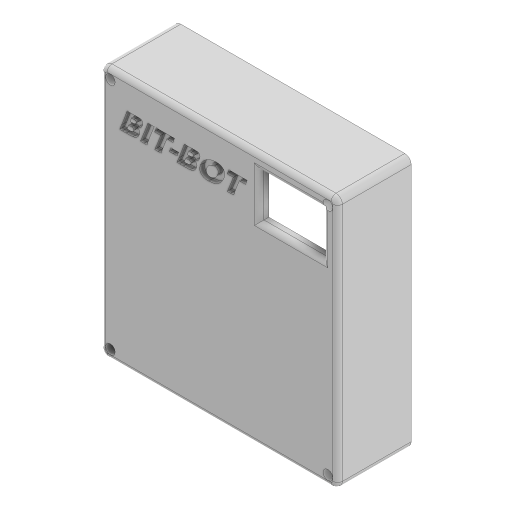
# Autodesk Inventor part: bit bot battery pack
Saved by Autodesk Inventor 2024 (Build 280153000, 153)
## iProperties
Created: 2024-01-11
Part Number: bit bot battery pack
Material: Generic
Document SubType Name: Modeling
Designer: chris
Density: 1 g/cm^3
Appearance: Default
Author: chris
Autodesk Inventor part; units mm, degrees
ref_plane "YZ Plane" through (0, 0, 0) normal (1, 0, 0) x (0, 1, 0)
ref_plane "XZ Plane" through (0, 0, 0) normal (0, 1, 0) x (-1, 0, 0)
ref_plane "XY Plane" through (0, 0, 0) normal (0, 0, 1) x (1, 0, 0)
sketch "Sketch2" plane through (0, 0, 0) normal (0, 0, 1) x (1, 0, 0)
  line L0 (0, -40) -> (0, -15)
  line L1 (0, -15) -> (-34, -15)
  line L2 (-34, -15) -> (-34, 58)
  line L3 (-34, 58) -> (34, 58)
  line L4 (34, 58) -> (34, -15)
  line L5 (34, -15) -> (0, -15)
  circle A0 centre (-34, 58) radius 1.5
  circle A1 centre (34, 58) radius 1.5
  circle A2 centre (-34, -15) radius 1.5
  circle A3 centre (34, -15) radius 1.5
  line L6 (32.5, 56.5) -> (-32.5, 56.5)
  line L7 (-32.5, 56.5) -> (-32.5, -13.5)
  line L8 (-32.5, -13.5) -> (0, -13.5)
  line L9 (0, -13.5) -> (32.5, -13.5)
  line L10 (32.5, -13.5) -> (32.5, 56.5)
  line L11 (37, -18) -> (37, 61)
  line L12 (37, 61) -> (-37, 61)
  line L13 (-37, 61) -> (-37, -18)
  line L14 (-37, -18) -> (0, -18)
  line L15 (0, -18) -> (37, -18)
  point P0 (0, 0)
  dimension "d0" = 25
  dimension "d1" = 34
  dimension "d3" = 68
  dimension "d4" = 3
  dimension "d5" = 3
  dimension "d6" = 3
  dimension "d11" = 1.5
  dimension "d13" = 3
  constraints: 32 end point, 13 perpendicular, 4 centre point, 4 coincident, 1 point on line, 1 vertical, 8 other
  measures "d0" distance of L0.start L0.end
  measures "d1" distance of L0.end L1.end
  measures "d3" distance of L2.end L3.end
  measures "d4" diameter of A0
  measures "d5" diameter of A1
  measures "d6" diameter of A2
  measures "d11" distance between parallel lines of L3 L6
  measures "d13" distance between parallel lines of L4 L11
extrude "Extrusion1" add sketch "Sketch2" along normal blind 20 contours L1 A2 L2 A0 L3 A1 L4 A3 L5 | L15 L14 L13 L12 L11
fillet "Fillet1" radius 2 4 edges at (37, -18, 10) (37, 61, 10) (-37, 61, 10) (-37, -18, 10)
sketch "Sketch3" plane through (0, 0, 20) normal (0, 0, 1) x (1, 0, 0)
  arc A0 (-37, -16) -> (-35, -18) centre (-35, -16) ccw projected
  line L0 (-35, -18) -> (35, -18) projected
  arc A1 (35, -18) -> (37, -16) centre (35, -16) ccw projected
  line L1 (37, -16) -> (37, 59) projected
  arc A2 (37, 59) -> (35, 61) centre (35, 59) ccw projected
  line L2 (35, 61) -> (-35, 61) projected
  arc A3 (-35, 61) -> (-37, 59) centre (-35, 59) ccw projected
  line L3 (-37, 59) -> (-37, -16) projected
  circle A4 centre (34, -15) radius 1.5 projected
  circle A5 centre (-34, -15) radius 1.5 projected
  circle A6 centre (-34, 58) radius 1.5 projected
  line L4 (32.5, 56.5) -> (32.5, -13.5) projected
  line L5 (32.5, -13.5) -> (-32.5, -13.5) projected
  line L6 (-32.5, -13.5) -> (-32.5, 56.5) projected
  line L7 (-32.5, 56.5) -> (32.5, 56.5) projected
  circle A7 centre (34, 58) radius 1.5 projected
  point P0 (0, 0)
extrude "Extrusion2" add sketch "Sketch3" along normal blind 3 contours L3 A3 L2 A2 L1 A1 L0 A0 | L4 L5 L6 L7
fillet "Fillet2" radius 1.5 8 edges at (36.4142, 60.4142, 23) (0, 61, 23) (-36.4142, 60.4142, 23) (-37, 21.5, 23) (-36.4142, -17.4142, 23) (0, -18, 23) (36.4142, -17.4142, 23) (37, 21.5, 23)
sketch "Sketch4" plane through (0, 0, 20) normal (0, 0, -1) x (-1, 0, 0)
  line L0 (-32.5, 56.5) -> (-32.5, -13.5) projected
  line L1 (-32.5, 56.5) -> (-12.5, 56.5)
  line L2 (32.5, 56.5) -> (-32.5, 56.5) projected
  line L3 (-12.5, 56.5) -> (-12.5, 42.5)
  line L4 (-12.5, 42.5) -> (-32.5, 42.5)
  point P0 (0, 0)
  dimension "d18" = 20
  dimension "d19" = 14
  constraints: 6 end point, 2 perpendicular, 1 point on line
  measures "d18" distance of L0.start L1.end
  measures "d19" distance of L1.end L3.end
extrude "Extrusion3" cut sketch "Sketch4" against normal blind 3
fillet "Fillet3" radius 1.5 4 edges at (12.5, 49.5, 23) (22.5, 56.5, 23) (32.5, 49.5, 23) (22.5, 42.5, 23)
sketch "Sketch7" plane through (0, 0, 0) normal (0, 0, -1) x (-1, 0, 0)
  line L0 (32.5, -13.5) -> (32.5, 56.5) projected
  line L1 (32.5, 56.5) -> (27.5, 56.5)
  line L2 (32.5, 56.5) -> (-32.5, 56.5) projected
  line L3 (27.5, 56.5) -> (29.5, 56.5)
  line L4 (29.5, 56.5) -> (29.5, 58.5)
  line L5 (29.5, 58.5) -> (25.5, 58.5)
  line L6 (25.5, 58.5) -> (25.5, 56.5)
  line L7 (29.5, 58.5) -> (31, 58.5)
  line L8 (31, 58.5) -> (31, 56.5)
  line L9 (25.5, 58.5) -> (24, 58.5)
  line L10 (24, 58.5) -> (24, 56.5)
  line L11 (0, 56.5) -> (0, 48.9008)
  line L12 (-32.5, 56.5) -> (-27.5, 56.5)
  line L13 (-32.5, 56.5) -> (32.5, 56.5)
  line L14 (-27.5, 56.5) -> (-29.5, 56.5)
  line L15 (-29.5, 56.5) -> (-29.5, 58.5)
  line L16 (-29.5, 58.5) -> (-25.5, 58.5)
  line L17 (-25.5, 58.5) -> (-25.5, 56.5)
  line L18 (-29.5, 58.5) -> (-31, 58.5)
  line L19 (-31, 58.5) -> (-31, 56.5)
  line L20 (-25.5, 58.5) -> (-24, 58.5)
  line L21 (-24, 58.5) -> (-24, 56.5)
  line L22 (24, 58.5) -> (-24, 58.5)
  point P0 (0, 0)
  dimension "d44" = 5
  dimension "d45" = 2
  dimension "d46" = 2
  dimension "d47" = 4
  dimension "d48" = 1.5
  dimension "d49" = 1.5
  constraints: 42 end point, 14 point on line, 11 symmetric about line, 4 perpendicular, 2 vertical, 1 midpoint, 1 parallel
  measures "d44" distance of L0.end L1.end
  measures "d45" distance of L1.end L3.end
  measures "d46" distance of L3.end L4.end
  measures "d47" distance of L4.end L5.end
  measures "d48" distance of L4.end L7.end
  measures "d49" distance of L5.end L9.end
extrude "Extrusion6" cut sketch "Sketch7" against normal up to surface (20 mm away)
fillet "Fillet5" radius 1.5 4 edges at (31, 58.5, 10) (31, 56.5, 10) (-31, 58.5, 10) (-31, 56.5, 10)
sketch "Sketch12" plane through (-35, -18, 0) normal (0, -1, 0) x (1, 0, 0)
  line L0 (1, 23) -> (69, 23) projected
  line L1 (35, 11.5) -> (17.5, 11.5)
  line L2 (17.5, 11.5) -> (52.5, 11.5)
  circle A0 centre (17.5, 11.5) radius 6
  circle A1 centre (52.5, 11.5) radius 6
  line L3 (35, 11.5) -> (35, 13)
  line L4 (35, 13) -> (17.5, 13)
  line L5 (17.5, 13) -> (53.6469, 13)
  line L6 (35, 11.5) -> (35, 10)
  line L7 (35, 10) -> (18.6171, 10)
  line L8 (18.6171, 10) -> (53.6469, 10)
  point P0 (35, 0)
  dimension "d60" = 17.5
  dimension "d61" = 35
  dimension "d62" = 12
  dimension "d63" = 12
  dimension "d68" = 1.5
  dimension "d69" = 1.5
  constraints: 16 end point, 3 perpendicular, 3 point on line, 2 centre point, 2 coincident, 1 horizontal, 1 vertical
  measures "d60" distance of L1.start L1.end
  measures "d61" distance of L1.end L2.end
  measures "d62" diameter of A0
  measures "d63" diameter of A1
  measures "d68" distance of L1.start L3.end
  measures "d69" distance of L1.start L6.end
extrude "Extrusion8" cut sketch "Sketch12" against normal blind 1 contours A0 | A1
sketch "Sketch13" plane through (0, 0, 23) normal (0, 0, 1) x (1, 0, 0)
  line L0 (-31.5692, 52.222) -> (-1.4752, 52.222) construction
  line L1 (-1.4752, 52.222) -> (-1.4752, 34.913) construction
  line L2 (-1.4752, 34.913) -> (-31.5692, 34.913) construction
  line L3 (-31.5692, 34.913) -> (-31.5692, 52.222) construction
  spline S0 degree 2 poles (-31.1035, 46.0094) (-30.6737, 46.992) (-30.4536, 47.5549) knots 0 0 0 1 1 1
  spline S1 degree 2 poles (-30.4536, 47.5549) (-30.1466, 48.3225) (-29.1487, 51.004) (-28.9593, 51.5567) knots 0 0 0 1 2 2 2
  spline S2 degree 2 poles (-28.9593, 51.5567) (-28.8928, 51.7512) (-28.7751, 52.1094) knots 0 0 0 1 1 1
  spline S3 degree 2 poles (-28.7751, 52.1094) (-28.1866, 52.0941) (-27.8386, 52.0941) knots 0 0 0 1 1 1
  spline S4 degree 2 poles (-27.8386, 52.0941) (-27.3525, 52.0941) (-26.0424, 52.135) (-25.5767, 52.135) knots 0 0 0 1 2 2 2
  spline S5 degree 2 poles (-25.5767, 52.135) (-25.0189, 52.135) (-24.7937, 52.1043) knots 0 0 0 1 1 1
  spline S6 degree 2 poles (-24.7937, 52.1043) (-24.4918, 52.0634) (-24.0926, 51.8587) (-23.9903, 51.7051) knots 0 0 0 1 2 2 2
  spline S7 degree 2 poles (-23.9903, 51.7051) (-23.8726, 51.5311) (-23.8624, 51.2804) knots 0 0 0 1 1 1
  spline S8 degree 2 poles (-23.8624, 51.2804) (-23.847, 50.9938) (-23.9596, 50.6663) knots 0 0 0 1 1 1
  spline S9 degree 2 poles (-23.9596, 50.6663) (-24.0466, 50.4104) (-24.3332, 49.9499) (-24.6914, 49.5865) (-25.0701, 49.346) (-25.3976, 49.2129) (-25.6586, 49.1464) knots 0 0 0 1 2 3 4 5 5 5
  spline S10 degree 2 poles (-25.6586, 49.1464) (-25.4334, 49.1055) (-25.1827, 49.0031) (-24.9319, 48.7728) (-24.7988, 48.4146) (-24.8193, 47.9745) (-24.9012, 47.7289) knots 0 0 0 1 2 3 4 5 5 5
  spline S11 degree 2 poles (-24.9012, 47.7289) (-25.0189, 47.386) (-25.4436, 46.7873) (-25.72, 46.5723) knots 0 0 0 1 2 2 2
  spline S12 degree 2 poles (-25.72, 46.5723) (-25.9503, 46.3881) (-26.5848, 46.1322) (-26.8868, 46.0811) knots 0 0 0 1 2 2 2
  spline S13 degree 2 poles (-26.8868, 46.0811) (-27.1324, 46.0452) (-28.3708, 46.0094) (-29.0617, 46.0094) knots 0 0 0 1 2 2 2
  line L4 (-29.0617, 46.0094) -> (-30.2336, 46.0145)
  line L5 (-30.2336, 46.0145) -> (-31.1035, 46.0094)
  line L6 (-28.8007, 47.2325) -> (-27.941, 47.2325)
  spline S14 degree 2 poles (-27.941, 47.2325) (-27.5981, 47.2325) (-27.4241, 47.2734) knots 0 0 0 1 1 1
  spline S15 degree 2 poles (-27.4241, 47.2734) (-27.2143, 47.3246) (-26.9533, 47.4832) (-26.7384, 47.7596) (-26.6769, 47.9336) knots 0 0 0 1 2 3 3 3
  spline S16 degree 2 poles (-26.6769, 47.9336) (-26.6309, 48.0769) (-26.6514, 48.302) (-26.7947, 48.4556) (-27.0608, 48.5221) (-27.3627, 48.5221) knots 0 0 0 1 2 3 4 4 4
  line L7 (-27.3627, 48.5221) -> (-28.3043, 48.5221)
  line L8 (-28.3043, 48.5221) -> (-28.8007, 47.2325)
  line L9 (-27.8488, 49.7349) -> (-27.2092, 49.7349)
  spline S17 degree 2 poles (-27.2092, 49.7349) (-26.897, 49.7349) (-26.6207, 49.7656) (-26.3443, 49.8475) (-26.0987, 50.0368) (-25.94, 50.2671) (-25.9042, 50.3848) knots 0 0 0 1 2 3 4 5 5 5
  spline S18 degree 2 poles (-25.9042, 50.3848) (-25.8479, 50.5486) (-25.9144, 50.8096) (-26.2215, 50.9324) (-26.5797, 50.9324) knots 0 0 0 1 2 3 3 3
  line L10 (-26.5797, 50.9324) -> (-27.3832, 50.9324)
  line L11 (-27.3832, 50.9324) -> (-27.8488, 49.7349)
  spline S19 degree 2 poles (-24.6095, 46.0094) (-23.1306, 49.5967) (-22.4755, 51.5311) knots 0 0 0 1 1 1
  line L12 (-22.4755, 51.5311) -> (-22.2811, 52.1094)
  spline S20 degree 2 poles (-22.2811, 52.1094) (-21.5032, 52.0992) (-21.2371, 52.0992) knots 0 0 0 1 1 1
  spline S21 degree 2 poles (-21.2371, 52.0992) (-21.1194, 52.0992) (-20.275, 52.1094) knots 0 0 0 1 1 1
  spline S22 degree 2 poles (-20.275, 52.1094) (-20.6998, 51.1064) (-21.0529, 50.2057) knots 0 0 0 1 1 1
  spline S23 degree 2 poles (-21.0529, 50.2057) (-21.5441, 48.9519) (-22.3374, 46.777) (-22.5983, 46.0094) knots 0 0 0 1 2 2 2
  line L13 (-22.5983, 46.0094) -> (-23.5092, 46.0196)
  spline S24 degree 2 poles (-23.5092, 46.0196) (-23.7754, 46.0196) (-24.6095, 46.0094) knots 0 0 0 1 1 1
  spline S25 degree 2 poles (-20.142, 46.0094) (-19.1799, 48.1792) (-18.2485, 50.7891) knots 0 0 0 1 1 1
  line L14 (-18.2485, 50.7891) -> (-20.1727, 50.7379)
  line L15 (-20.1727, 50.7379) -> (-19.9782, 51.2343)
  spline S26 degree 2 poles (-19.9782, 51.2343) (-19.8247, 51.6335) (-19.6558, 52.1094) knots 0 0 0 1 1 1
  spline S27 degree 2 poles (-19.6558, 52.1094) (-18.3918, 52.0992) (-16.703, 52.0992) knots 0 0 0 1 1 1
  line L16 (-16.703, 52.0992) -> (-15.5977, 52.1043)
  line L17 (-15.5977, 52.1043) -> (-14.523, 52.1043)
  line L18 (-14.523, 52.1043) -> (-13.9396, 52.1094)
  line L19 (-13.9396, 52.1094) -> (-14.1187, 51.6693)
  spline S28 degree 2 poles (-14.1187, 51.6693) (-14.2569, 51.3162) (-14.4258, 50.8556) (-14.4667, 50.7379) knots 0 0 0 1 2 2 2
  spline S29 degree 2 poles (-14.4667, 50.7379) (-15.4032, 50.7891) (-16.0224, 50.7891) knots 0 0 0 1 1 1
  line L20 (-16.0224, 50.7891) -> (-16.3397, 50.7891)
  spline S30 degree 2 poles (-16.3397, 50.7891) (-16.6723, 50.001) (-16.9384, 49.3306) knots 0 0 0 1 1 1
  spline S31 degree 2 poles (-16.9384, 49.3306) (-17.312, 48.3737) (-17.9773, 46.5672) (-18.1666, 46.0094) knots 0 0 0 1 2 2 2
  spline S32 degree 2 poles (-18.1666, 46.0094) (-18.8984, 46.0196) (-19.1134, 46.0196) knots 0 0 0 1 1 1
  spline S33 degree 2 poles (-19.1134, 46.0196) (-19.3027, 46.0196) (-20.142, 46.0094) knots 0 0 0 1 1 1
  spline S34 degree 2 poles (-15.5618, 47.7545) (-15.2855, 48.4095) (-15.0706, 49.0031) knots 0 0 0 1 1 1
  spline S35 degree 2 poles (-15.0706, 49.0031) (-14.4411, 48.9827) (-13.8782, 48.9827) knots 0 0 0 1 1 1
  spline S36 degree 2 poles (-13.8782, 48.9827) (-13.3102, 48.9827) (-12.6705, 49.0031) knots 0 0 0 1 1 1
  spline S37 degree 2 poles (-12.6705, 49.0031) (-12.9212, 48.4197) (-13.1618, 47.7545) knots 0 0 0 1 1 1
  spline S38 degree 2 poles (-13.1618, 47.7545) (-13.7912, 47.7698) (-14.3592, 47.7698) knots 0 0 0 1 1 1
  spline S39 degree 2 poles (-14.3592, 47.7698) (-14.9273, 47.7698) (-15.5618, 47.7545) knots 0 0 0 1 1 1
  spline S40 degree 2 poles (-13.2283, 46.0094) (-12.7984, 46.992) (-12.5784, 47.5549) knots 0 0 0 1 1 1
  spline S41 degree 2 poles (-12.5784, 47.5549) (-12.2713, 48.3225) (-11.2734, 51.004) (-11.0841, 51.5567) knots 0 0 0 1 2 2 2
  spline S42 degree 2 poles (-11.0841, 51.5567) (-11.0176, 51.7512) (-10.8999, 52.1094) knots 0 0 0 1 1 1
  spline S43 degree 2 poles (-10.8999, 52.1094) (-10.3113, 52.0941) (-9.9634, 52.0941) knots 0 0 0 1 1 1
  spline S44 degree 2 poles (-9.9634, 52.0941) (-9.4772, 52.0941) (-8.1671, 52.135) (-7.7014, 52.135) knots 0 0 0 1 2 2 2
  spline S45 degree 2 poles (-7.7014, 52.135) (-7.1436, 52.135) (-6.9185, 52.1043) knots 0 0 0 1 1 1
  spline S46 degree 2 poles (-6.9185, 52.1043) (-6.6165, 52.0634) (-6.2174, 51.8587) (-6.115, 51.7051) knots 0 0 0 1 2 2 2
  spline S47 degree 2 poles (-6.115, 51.7051) (-5.9973, 51.5311) (-5.9871, 51.2804) knots 0 0 0 1 1 1
  spline S48 degree 2 poles (-5.9871, 51.2804) (-5.9717, 50.9938) (-6.0843, 50.6663) knots 0 0 0 1 1 1
  spline S49 degree 2 poles (-6.0843, 50.6663) (-6.1713, 50.4104) (-6.4579, 49.9499) (-6.8161, 49.5865) (-7.1948, 49.346) (-7.5223, 49.2129) (-7.7833, 49.1464) knots 0 0 0 1 2 3 4 5 5 5
  spline S50 degree 2 poles (-7.7833, 49.1464) (-7.5582, 49.1055) (-7.3074, 49.0031) (-7.0566, 48.7728) (-6.9236, 48.4146) (-6.9441, 47.9745) (-7.0259, 47.7289) knots 0 0 0 1 2 3 4 5 5 5
  spline S51 degree 2 poles (-7.0259, 47.7289) (-7.1436, 47.386) (-7.5684, 46.7873) (-7.8447, 46.5723) knots 0 0 0 1 2 2 2
  spline S52 degree 2 poles (-7.8447, 46.5723) (-8.075, 46.3881) (-8.7096, 46.1322) (-9.0115, 46.0811) knots 0 0 0 1 2 2 2
  spline S53 degree 2 poles (-9.0115, 46.0811) (-9.2572, 46.0452) (-10.4956, 46.0094) (-11.1864, 46.0094) knots 0 0 0 1 2 2 2
  line L21 (-11.1864, 46.0094) -> (-12.3583, 46.0145)
  line L22 (-12.3583, 46.0145) -> (-13.2283, 46.0094)
  line L23 (-10.9254, 47.2325) -> (-10.0657, 47.2325)
  spline S54 degree 2 poles (-10.0657, 47.2325) (-9.7228, 47.2325) (-9.5488, 47.2734) knots 0 0 0 1 1 1
  spline S55 degree 2 poles (-9.5488, 47.2734) (-9.339, 47.3246) (-9.078, 47.4832) (-8.8631, 47.7596) (-8.8017, 47.9336) knots 0 0 0 1 2 3 3 3
  spline S56 degree 2 poles (-8.8017, 47.9336) (-8.7556, 48.0769) (-8.7761, 48.302) (-8.9194, 48.4556) (-9.1855, 48.5221) (-9.4874, 48.5221) knots 0 0 0 1 2 3 4 4 4
  line L24 (-9.4874, 48.5221) -> (-10.429, 48.5221)
  line L25 (-10.429, 48.5221) -> (-10.9254, 47.2325)
  line L26 (-9.9736, 49.7349) -> (-9.3339, 49.7349)
  spline S57 degree 2 poles (-9.3339, 49.7349) (-9.0217, 49.7349) (-8.7454, 49.7656) (-8.4691, 49.8475) (-8.2234, 50.0368) (-8.0648, 50.2671) (-8.029, 50.3848) knots 0 0 0 1 2 3 4 5 5 5
  spline S58 degree 2 poles (-8.029, 50.3848) (-7.9727, 50.5486) (-8.0392, 50.8096) (-8.3462, 50.9324) (-8.7045, 50.9324) knots 0 0 0 1 2 3 3 3
  line L27 (-8.7045, 50.9324) -> (-9.5079, 50.9324)
  line L28 (-9.5079, 50.9324) -> (-9.9736, 49.7349)
  spline S59 degree 2 poles (-0.9464, 52.222) (-0.2351, 52.222) (0.9573, 51.8382) (1.6635, 50.9938) (1.7812, 49.8936) (1.5407, 49.1822) knots 0 0 0 1 2 3 4 4 4
  spline S60 degree 2 poles (1.5407, 49.1822) (1.2848, 48.43) (0.3176, 47.1762) (-1.0027, 46.296) (-2.5482, 45.8917) (-3.3158, 45.8917) knots 0 0 0 1 2 3 4 4 4
  spline S61 degree 2 poles (-3.3158, 45.8917) (-4.0681, 45.8917) (-5.3218, 46.2909) (-6.0434, 47.1762) (-6.0997, 48.2662) (-5.8745, 48.9366) knots 0 0 0 1 2 3 4 4 4
  spline S62 degree 2 poles (-5.8745, 48.9366) (-5.5419, 49.914) (-4.1295, 51.393) (-2.0671, 52.222) (-0.9464, 52.222) knots 0 0 0 1 2 3 3 3
  spline S63 degree 2 poles (-1.4889, 50.8761) (-2.0006, 50.8761) (-3.0036, 50.3695) (-3.7559, 49.4739) (-3.9299, 48.9622) knots 0 0 0 1 2 3 3 3
  spline S64 degree 2 poles (-3.9299, 48.9622) (-4.0885, 48.4863) (-3.9504, 47.6982) (-3.2697, 47.2581) (-2.804, 47.2581) knots 0 0 0 1 2 3 3 3
  spline S65 degree 2 poles (-2.804, 47.2581) (-2.3077, 47.2581) (-1.3149, 47.7545) (-0.578, 48.65) (-0.4091, 49.1413) knots 0 0 0 1 2 3 3 3
  spline S66 degree 2 poles (-0.4091, 49.1413) (-0.2453, 49.6223) (-0.3733, 50.4309) (-0.9976, 50.8761) (-1.4889, 50.8761) knots 0 0 0 1 2 3 3 3
  spline S67 degree 2 poles (2.5335, 46.0094) (3.4955, 48.1792) (4.4269, 50.7891) knots 0 0 0 1 1 1
  line L29 (4.4269, 50.7891) -> (2.5027, 50.7379)
  line L30 (2.5027, 50.7379) -> (2.6972, 51.2343)
  spline S68 degree 2 poles (2.6972, 51.2343) (2.8507, 51.6335) (3.0196, 52.1094) knots 0 0 0 1 1 1
  spline S69 degree 2 poles (3.0196, 52.1094) (4.2836, 52.0992) (5.9724, 52.0992) knots 0 0 0 1 1 1
  line L31 (5.9724, 52.0992) -> (7.0777, 52.1043)
  line L32 (7.0777, 52.1043) -> (8.1524, 52.1043)
  line L33 (8.1524, 52.1043) -> (8.7358, 52.1094)
  line L34 (8.7358, 52.1094) -> (8.5567, 51.6693)
  spline S70 degree 2 poles (8.5567, 51.6693) (8.4185, 51.3162) (8.2496, 50.8556) (8.2087, 50.7379) knots 0 0 0 1 2 2 2
  spline S71 degree 2 poles (8.2087, 50.7379) (7.2722, 50.7891) (6.653, 50.7891) knots 0 0 0 1 1 1
  line L35 (6.653, 50.7891) -> (6.3357, 50.7891)
  spline S72 degree 2 poles (6.3357, 50.7891) (6.0031, 50.001) (5.737, 49.3306) knots 0 0 0 1 1 1
  spline S73 degree 2 poles (5.737, 49.3306) (5.3634, 48.3737) (4.6981, 46.5672) (4.5088, 46.0094) knots 0 0 0 1 2 2 2
  spline S74 degree 2 poles (4.5088, 46.0094) (3.777, 46.0196) (3.5621, 46.0196) knots 0 0 0 1 1 1
  spline S75 degree 2 poles (3.5621, 46.0196) (3.3727, 46.0196) (2.5335, 46.0094) knots 0 0 0 1 1 1
  point P0 (0, 0)
  constraints: 2 other
extrude "Extrusion9" cut sketch "Sketch13" against normal blind 1.5
body "Solid1"
